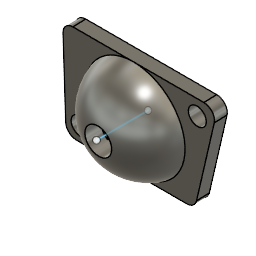
_Z Arm Copy_Component2.59cd4705-7b90-461e-99cb-14aab5ead7ad (Autodesk Fusion 360 design; units mm, degrees)
Autodesk Fusion 360 part; units mm, degrees
sketch "Sketch1" plane through (0, -4.9412, 145.9698) normal (0, -0.033831, 0.999428) x (1, 0, 0)
  line L0 (164.9167, 8.258) -> (193.6585, 119.5797)
  line L1 (193.6585, 119.5797) -> (156.6913, 119.5797)
  line L2 (156.6913, 119.5797) -> (156.6913, 8.258)
  line L3 (156.6913, 8.258) -> (164.9167, 8.258)
  line L4 (156.6913, 92.5946) -> (186.6913, 92.5946)
  line L5 (156.6913, 73.2288) -> (181.6913, 73.2288)
  line L6 (171.6913, 92.5946) -> (169.1913, 73.2288) construction
  circle A0 centre (170.4413, 82.9117) radius 2.6
  circle A1 centre (170.4413, 82.9117) radius 1.15
  line L7 (173.0413, 82.9117) -> (169.0413, 82.9117) construction
  line L8 (169.0413, 85.1026) -> (169.0413, 80.7208)
  line L9 (186.6913, 92.5946) -> (181.6913, 73.2288)
  line L10 (156.6913, 92.5946) -> (156.6913, 73.2288)
  circle A2 centre (170.4413, 82.9117) radius 7
  dimension "d1" = 30
  dimension "d2" = 25
  dimension "d3" = 5.2
  dimension "d4" = 2.3
  dimension "d5" = 4
  dimension "d6" = 14
  constraint coincident L2 L4.start
  constraint coincident L0 L4.end
  constraint perpendicular L2 L4
  constraint coincident L2 L5.start
  constraint coincident L0 L5.end
  constraint perpendicular L2 L5
  constraint midpoint L4 L6.start
  constraint midpoint L5 L6.end
  constraint midpoint L6 A0.centre
  constraint concentric A0 A1
  constraint coincident A0 L7.start
  constraint horizontal L7
  constraint coincident A0 L8.start
  constraint perpendicular L7 L8
  constraint coincident A0 L8.end
  constraint concentric A1 A2
  measures "d1" distance of L4.start L4.end
  measures "d2" distance of L5.start L5.end
  measures "d3" diameter of A0
  measures "d4" diameter of A1
  measures "d5" distance of L7.start L7.end
  measures "d6" diameter of A2
sketch "Sketch2" plane through (0, -5.0258, 148.4683) normal (0, -0.033831, 0.999428) x (1, 0, 0)
  arc A0 (180.1421, 73.2288) -> (182.0786, 74.7288) centre (180.1421, 75.2288) ccw
  line L0 (182.0786, 74.7288) -> (186.0458, 90.0946)
  arc A1 (186.0458, 90.0946) -> (184.1093, 92.5946) centre (184.1093, 90.5946) ccw
  line L1 (184.1093, 92.5946) -> (158.6913, 92.5946)
  arc A2 (158.6913, 92.5946) -> (156.6913, 90.5946) centre (158.6913, 90.5946) ccw
  line L2 (156.6913, 90.5946) -> (156.6913, 75.2288)
  arc A3 (156.6913, 75.2288) -> (158.6913, 73.2288) centre (158.6913, 75.2288) ccw
  line L3 (158.6913, 73.2288) -> (180.1421, 73.2288)
  circle A4 centre (170.4413, 82.9117) radius 9.6825
  line L4 (156.6913, 73.2288) -> (159.5197, 76.0572)
  line L5 (156.6913, 73.2288) -> (160.6913, 73.2288) construction
  circle A5 centre (159.5197, 76.0572) radius 1.75
  line L6 (186.6913, 92.5946) -> (182.7379, 89.5335)
  line L7 (186.6913, 92.5946) -> (191.6913, 92.5946) construction
  circle A6 centre (182.7379, 89.5335) radius 1.75
  dimension "d7" = 45
  dimension "d8" = 4
  dimension "d9" = 3.5
  dimension "d25" = 142.25
  dimension "d26" = 5
  dimension "d27" = 3.5
  constraint horizontal L5
  constraint coincident L4.end A5.centre
  constraint horizontal L7
  constraint coincident L6.end A6.centre
  measures "d7" angle of L4 L5
  measures "d8" distance of L4.start L4.end
  measures "d9" diameter of A5
  measures "d25" angle of L6 L7
  measures "d26" distance of L6.start L6.end
  measures "d27" diameter of A6
sketch "Sketch3" plane through (0, 77.923, 0) normal (0, 1, 0) x (1, 0, 0)
  line L0 (170.4413, -148.7748) -> (170.4413, -158.7748)
  arc A0 (160.4413, -148.7748) -> (170.4413, -158.7748) centre (170.4413, -148.7748) ccw
  line L1 (170.4413, -148.7748) -> (160.4413, -148.7748)
  point P0 (170.4413, -148.7748)
  dimension "d28" = 20
  constraint coincident P0 L0.start
  measures "d28" diameter of A0
revolve "Revolve1" add sketch "Sketch3" angle 360 about axis through (170.4413, 77.923, 148.7748) along (0, 0, 1)
extrude "Extrude1" add sketch "Sketch1" along normal blind 2.5 contours L0 L2 L4 L5 L9 L10 | A2
delete_face "DeleteFace1" 1 faces at (169.4995, 87.8331, 149.7254)
delete_face "DeleteFace2" 1 faces at (169.5783, 77.7207, 148.7748)
extrude "Extrude2" cut sketch "Sketch1" along normal blind 12 contours A1
delete_face "DeleteFace3" 1 faces at (171.4105, 67.9968, 149.503)
extrude "Extrude3" cut sketch "Sketch1" along normal blind 15 from surface at 5 contours A0 L8 | A0 L8
extrude "Extrude4" add sketch "Sketch1" along normal blind 1.5 from surface at 5 contours A0 L8 picked at (168.7796, 82.4421)
extrude "Extrude5" cut sketch "Sketch1" along normal blind 2 contours A0 L8 | A0 L8
fillet "Fillet1" radius 2 4 edges at (186.6913, 87.5581, 150.3517) (156.6913, 87.5581, 150.3517) (156.6913, 68.2034, 149.6965) (181.6913, 68.2034, 149.6965)
extrude "Extrude6" cut sketch "Sketch2" against normal blind 5 contours A5 | A6
